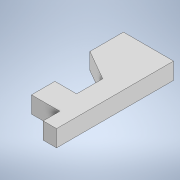
# Autodesk Inventor part: Practica3
Saved by Autodesk Inventor 2020 (Build 240168000, 168)
## iProperties
Created: 2020-02-12
Part Number: Practica3
Material: Genérico
Document SubType Name: Chapa
Designer: luisg
Density: 1 g/cm^3
Sheet Metal Rule: Por defecto_mm
Appearance: Valor por defecto
Author: luisg
Autodesk Inventor part; units mm, degrees
ref_plane "YZ Plane" through (0, 0, 0) normal (1, 0, 0) x (0, 1, 0)
ref_plane "XZ Plane" through (0, 0, 0) normal (0, 1, 0) x (-1, 0, 0)
ref_plane "XY Plane" through (0, 0, 0) normal (0, 0, 1) x (1, 0, 0)
sketch "Boceto1" plane through (0, 0, 0) normal (0, 1, 0) x (-1, 0, 0)
  line L0 (0, 0) -> (0, -70)
  line L1 (0, -70) -> (30, -70)
  line L2 (30, -70) -> (30, -50)
  line L3 (30, -50) -> (12, -39.6077)
  line L4 (12, -24) -> (25, -24)
  line L5 (25, -24) -> (25, -10)
  line L6 (25, -10) -> (8, -10)
  line L7 (8, 0) -> (0, 0)
  line L8 (12, -24) -> (12, -39.6077)
  line L9 (8, -10) -> (8, 0)
  dimension "d0" = 20
  dimension "d1" = 70
  dimension "d2" = 30
  dimension "d5" = 25
  dimension "d6" = 10
  dimension "d7" = 8
  dimension "d8" = 12
  dimension "d9" = 120
  dimension "d10" = 14
  constraints: 20 end point, 5 perpendicular, 2 vertical
  measures "d0" distance of L1.end L2.end
  measures "d1" distance of L0.start L0.end
  measures "d2" distance of L0.end L1.end
  measures "d5" distance between parallel lines of L0 L5
  measures "d6" distance between parallel lines of L6 L7
  measures "d7" distance between parallel lines of L0 L9
  measures "d8" distance between parallel lines of L0 L8
  measures "d9" angle of L8 L3
  measures "d10" distance of L4.end L5.end
extrude "Extrusión1" add sketch "Boceto1" along normal blind 10
equation "\"Radio_pliegue\" = Grosor"
equation "\"Anchura_desahogo_plegado\" = Grosor"
equation "\"Profundidad_desahogo_plegado\" = 0.5 * Grosor"
equation "\"Tamaño_destalonado\" = 4 * Grosor"
equation "\"Remanente_mínimo\" = 2 * Grosor"
equation "\"Radiodetransición\" = Radio_pliegue"
equation "\"Tamaño_de_radio_de_Jacobi\" = Radio_pliegue"
equation "\"TamañoSeparación\" = Grosor"
equation "\"Grosor\" = 0.5"
